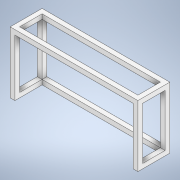
# Autodesk Inventor part: Goal
Saved by Autodesk Inventor 2022 (Build 260153000, 153)
## iProperties
Created: 2022-10-30
Part Number: Goal
Material: 一般
Document SubType Name: Modeling
Designer: Masato Kubotera
Density: 1 g/cm^3
Appearance: 既定
Author: Masato Kubotera
Autodesk Inventor part; units mm, degrees
ref_plane "YZ Plane" through (0, 0, 0) normal (1, 0, 0) x (0, 1, 0)
ref_plane "XZ Plane" through (0, 0, 0) normal (0, 1, 0) x (-1, 0, 0)
ref_plane "XY Plane" through (0, 0, 0) normal (0, 0, 1) x (1, 0, 0)
sketch "スケッチ1" plane through (0, 0, 0) normal (0, 0, 1) x (1, 0, 0)
  line L0 (-30, 130) -> (30, 130) construction
  line L1 (30, 130) -> (30, -130) construction
  line L2 (30, -130) -> (-30, -130) construction
  line L3 (-30, -130) -> (-30, 130) construction
  line L4 (-30, 130) -> (30, -130) construction
  line L5 (30, 130) -> (-30, -130) construction
  line L6 (35, 135) -> (-32.5, 135)
  line L7 (-32.5, 135) -> (-32.5, 125)
  line L8 (-32.5, 125) -> (-22.5, 125)
  line L9 (25, 125) -> (25, -125)
  line L10 (25, -125) -> (-22.5, -125)
  line L11 (-32.5, -125) -> (-32.5, -135)
  line L12 (-32.5, -135) -> (35, -135)
  line L13 (35, -135) -> (35, 135)
  line L14 (35, 0) -> (-30, 0) construction
  line L15 (-32.5, 125) -> (-32.5, -125)
  line L16 (-22.5, -135) -> (-22.5, -125)
  line L17 (25, 125) -> (25, 135)
  line L18 (25, -125) -> (25, -135)
  line L19 (25, -125) -> (35, -125)
  line L20 (25, 125) -> (35, 125)
  line L21 (-22.5, 125) -> (-22.5, 130)
  line L22 (-22.5, -125) -> (-22.5, 125)
  line L23 (-22.5, 130) -> (-22.5, 135)
  line L24 (-22.5, 125) -> (25, 125)
  line L25 (-22.5, -125) -> (-32.5, -125)
  point P0 (0, 0)
  point P1 (0, 0)
  point P2 (0, 0)
  dimension "d0" = 60
  dimension "d1" = 260
  dimension "d2" = 10
  dimension "d3" = 10
  dimension "d4" = 2.5
  dimension "d5" = 10
  constraints: 52 end point, 17 perpendicular, 8 point on line, 5 midpoint, 4 parallel, 2 horizontal, 1 coincident, 1 collinear, 5 other
  measures "d0" distance of L0.start L0.end
  measures "d1" distance of L2.end L0.start
  measures "d2" distance between parallel lines of L6 L8
  measures "d3" distance between parallel lines of L13 L9
  measures "d4" distance between parallel lines of L7 L3
  measures "d5" distance between parallel lines of L16 L15
extrude "押し出し1" add sketch "スケッチ1" along normal blind 130 contours L13 L20 L17 L6 | L17 L24 L21 L23 L6 | L13 L19 L9 L20 | L23 L21 L8 L7 L6 | L13 L12 L18 L19 | L18 L12 L16 L10 | L22 L25 L15 L8 | L16 L12 L11 L25
extrude "押し出し2" cut sketch "スケッチ1" along normal blind 120 contours L17 L24 L21 L23 L6 | L13 L19 L9 L20 | L9 L10 L22 L24 | L18 L12 L16 L10 | L22 L25 L15 L8
extrude "押し出し3" add sketch "スケッチ1" along normal blind 10 contours L17 L24 L21 L23 L6 | L13 L19 L9 L20 | L18 L12 L16 L10
equation "\"d3\" = d2"
equation "\"d5\" = d2"
